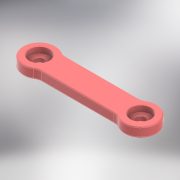
# Autodesk Inventor part: BRAÇO ROBÓTICO - Garra A2
Saved by Autodesk Inventor 2021 (Build 250183000, 183)
## iProperties
Created: 2020-08-23
Part Number: BRAÇO ROBÓTICO - Garra A2
Material: Plástico PC/ABS
Document SubType Name: Modeling
Designer: Araújo, I.
Mass: 0.160046 g
Surface Area: 6.28916 cm^2
Volume: 0.447966 cm^3
Density: 0.357273 g/cm^3
Appearance: Liso - Branco
Author: Araújo, I.
## iProperties of the stored document _3DPrint.ipt
Created: 2020-11-23
Part Number: _3DPrint
Material: Genérico
Document SubType Name: Modeling
Designer: Araújo, I.
Mass: 0.447966 g
Surface Area: 6.28916 cm^2
Volume: 0.447966 cm^3
Density: 1 g/cm^3
Appearance: Padrão
Author: Araújo, I.
Autodesk Inventor part; units mm, degrees
ref_plane "YZ Plane" through (0, 0, 0) normal (1, 0, 0) x (0, 1, 0)
ref_plane "XZ Plane" through (0, 0, 0) normal (0, 1, 0) x (-1, 0, 0)
ref_plane "XY Plane" through (0, 0, 0) normal (0, 0, 1) x (1, 0, 0)
sketch "Esboço1" plane through (0, 0, 0) normal (0, 1, 0) x (-1, 0, 0)
  circle A0 centre (0, 0) radius 1.25
  arc A1 (-2.0603, -3.4286) -> (-2.0603, 3.4286) centre (0, 0) ccw
  circle A2 centre (-25, 0) radius 1.25
  arc A3 (-22.9397, 3.4286) -> (-22.9397, -3.4286) centre (-25, 0) ccw
  line L0 (-3.6056, -3) -> (-21.3944, -3)
  line L1 (-3.6056, 3) -> (-21.3944, 3)
  arc A4 (-2.0603, -3.4286) -> (-3.6056, -3) centre (-3.6056, -6) ccw
  arc A5 (-3.6056, 3) -> (-2.0603, 3.4286) centre (-3.6056, 6) ccw
  arc A6 (-21.3944, -3) -> (-22.9397, -3.4286) centre (-21.3944, -6) ccw
  arc A7 (-22.9397, 3.4286) -> (-21.3944, 3) centre (-21.3944, 6) ccw
  point P0 (-2.6458, -3)
  point P1 (-22.3542, -3)
  point P2 (-2.6458, 3)
  point P3 (-22.3542, 3)
  dimension "d1" = 2.5
  dimension "d3" = 6
  dimension "d5" = 3
  dimension "d6" = 25
  dimension "d10" = 4
  constraints: 16 point on circle, 8 centre point, 8 tangent, 5 equal radius, 4 end point, 4 point on line, 3 coincident, 2 parallel, 1 horizontal, 1 horizontal alignment
  measures "d1" diameter of A0
  measures "d3" distance between parallel lines of L1 L0
  measures "d5" radius of A4
  measures "d6" distance of A2.centre A0.centre
  measures "d10" radius of A1
extrude "Extrusão1" add sketch "Esboço1" along normal blind 2.5
fillet "Arredondamento1" radius 0.3 16 edges at (22.1962, 0, 3.1091) (29, 0, 0) (22.1962, 0, -3.1091) (12.5, 0, -3) (2.8038, 0, -3.1091) (-4, 0, 0) (2.8038, 0, 3.1091) (12.5, 0, 3) (22.1962, 2.5, 3.1091) (29, 2.5, 0) (22.1962, 2.5, -3.1091) (12.5, 2.5, -3) (2.8038, 2.5, -3.1091) (-4, 2.5, 0) (2.8038, 2.5, 3.1091) (12.5, 2.5, 3)
sketch "Esboço2" plane through (0, 2.5, 0) normal (0, 1, 0) x (1, 0, 0)
  circle A0 centre (0, 0) radius 2.5
  circle A1 centre (25, 0) radius 1.25 projected
  circle A2 centre (25, 0) radius 2.5
  dimension "d11" = 5
  constraints: 2 centre point, 2 coincident, 1 equal radius
  measures "d11" diameter of A0
extrude "Extrusão2" cut sketch "Esboço2" against normal blind 1.5
